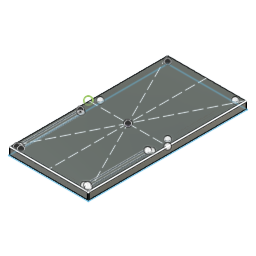
baseplate (Autodesk Fusion 360 design; units mm, degrees)
Autodesk Fusion 360 part; units mm, degrees
sketch "Sketch1" plane through (0, 0, 0) normal (0, 0, 1) x (1, 0, 0)
  line L0 (-50, 100) -> (50, 100)
  line L1 (50, 100) -> (50, -100)
  line L2 (50, -100) -> (-50, -100)
  line L3 (-50, -100) -> (-50, 100)
  dimension "d2" = 100
  dimension "d3" = 200
  constraint horizontal L0
  constraint vertical L1
  constraint horizontal L2
  constraint vertical L3
  measures "d2" distance of L0.start L0.end
  measures "d3" distance of L0.start L2.end
extrude "Extrude1" add sketch "Sketch1" along normal blind 10
sketch "Sketch2" plane through (0, 0, 10) normal (0, 0, 1) x (-1, 0, 0)
  line L0 (50, 100) -> (-50, 100)
  line L1 (-50, 100) -> (-50, -100)
  line L2 (-50, -100) -> (50, -100)
  line L3 (50, -100) -> (50, 100)
  line L4 (50, 0) -> (-50, 0) construction
  line L5 (0, -100) -> (0, 100) construction
  line L6 (50, -100) -> (-50, -100)
  line L7 (-50, -100) -> (-50, 100)
  line L8 (-50, 100) -> (50, 100)
  line L9 (50, 100) -> (50, -100)
  line L10 (50, -100) -> (-50, 100) construction
  line L11 (-50, -100) -> (50, 100) construction
  circle A0 centre (42.5, -92.5) radius 2.6
  circle A1 centre (-42.5, -92.5) radius 2.6
  circle A2 centre (42.5, -7.5) radius 2.6
  circle A3 centre (-42.5, -7.5) radius 2.6
  line L12 (43, 95) -> (41.8, 95)
  line L13 (39.8, 93) -> (39.8, 17)
  line L14 (41.8, 15) -> (43, 15)
  line L15 (45, 17) -> (45, 93)
  arc A4 (41.8, 95) -> (39.8, 93) centre (41.8, 93) ccw
  arc A5 (45, 93) -> (43, 95) centre (43, 93) ccw
  arc A6 (39.8, 17) -> (41.8, 15) centre (41.8, 17) ccw
  arc A7 (43, 15) -> (45, 17) centre (43, 17) ccw
  line L16 (-43, 95) -> (-41.8, 95)
  arc A8 (-45, 17) -> (-43, 15) centre (-43, 17) ccw
  line L17 (-41.8, 15) -> (-43, 15)
  arc A9 (-39.8, 93) -> (-41.8, 95) centre (-41.8, 93) ccw
  arc A10 (-41.8, 15) -> (-39.8, 17) centre (-41.8, 17) ccw
  line L18 (-39.8, 93) -> (-39.8, 17)
  arc A11 (-43, 95) -> (-45, 93) centre (-43, 93) ccw
  line L19 (-45, 17) -> (-45, 93)
  point P0 (42.5, -92.5)
  point P1 (45, 95)
  point P2 (39.8, 95)
  point P3 (45, 15)
  point P4 (-45, 95)
  point P5 (-39.8, 95)
  point P6 (-45, 15)
  dimension "d45" = 100
  dimension "d46" = 200
  dimension "d47" = 7.5
  dimension "d48" = 7.5
  dimension "d49" = 5.2
  dimension "d52" = -85
  dimension "d53" = 85
  dimension "d56" = 5.2
  dimension "d57" = 80
  dimension "d58" = 5
  dimension "d59" = 2
  dimension "d68" = 15
  constraint midpoint L4 origin
  constraint vertical L5
  constraint midpoint L2 L5.start
  constraint horizontal L6
  constraint perpendicular L6 L7
  constraint parallel L6 L8
  constraint parallel L7 L9
  constraint coincident L10 origin
  constraint coincident L11 origin
  constraint coincident P0 A0.centre
  constraint horizontal L12
  constraint vertical L13
  constraint horizontal L14
  constraint vertical L15
  constraint coincident P2 L12
  constraint coincident P2 L13
  constraint tangent L12 A4
  constraint tangent L13 A4
  constraint coincident P1 L12
  constraint coincident P1 L15
  constraint tangent L12 A5
  constraint tangent L15 A5
  constraint equal A4 A5
  constraint tangent L13 A6
  constraint tangent L14 A6
  constraint equal A4 A6
  constraint coincident P3 L14
  constraint coincident P3 L15
  constraint tangent L14 A7
  constraint tangent L15 A7
  constraint equal A4 A7
  constraint symmetric L5 P1 P4
  constraint symmetric L5 P2 P5
  constraint symmetric L5 P3 P6
  constraint symmetric L5 L12.end L16.end
  constraint symmetric L5 L13.start A9.start
  constraint symmetric L5 A4 A9
  constraint symmetric L5 L12.start L16.start
  constraint symmetric L5 L15.end A11.end
  constraint symmetric L5 A5 A11
  constraint symmetric L5 L13.end A10.end
  constraint symmetric L5 L14.start L17.start
  constraint symmetric L5 A6 A10
  constraint symmetric L5 L14.end A8.end
  constraint symmetric L5 L15.start A8.start
  constraint symmetric L5 A7 A8
  constraint midpoint L5.end L8
  measures "d45" distance of L0.end L0.start
  measures "d46" distance of L1.end L0.end
  measures "d47" distance of L6 P0
  measures "d48" distance of L9 P0
  measures "d49" diameter of A0
  measures "d56" distance of P1 P2
  measures "d57" distance of P1 P3
  measures "d58" distance of L9 L15
  measures "d59" radius of A4
  measures "d68" vertical distance of L4.start P3
extrude "Extrude4" cut sketch "Sketch2" against normal up to surface (10 mm away) contours L12 L13 L14 L15 A4 A5 A6 A7 | L16 A8 L17 A9 A10 L18 A11 L19
hole "Hole2" at (-42.5, 92.5, 10) at (42.5, 92.5, 10) at (42.5, 7.5, 10) at (-42.5, 7.5, 10) direction (0, 0, -1) diameter 5.2 end through all
fillet "Fillet3" radius 1 4 faces at (50, 33.3333, 3.3333) (16.6667, -100, 3.3333) (-50, -33.3333, 3.3333) (-16.6667, 100, 3.3333)
